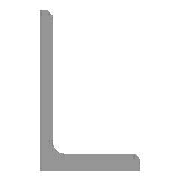
# Autodesk Inventor part: ISO 657-2 - 50x 30x 5-1448.59
Saved by Autodesk Inventor 2023 (Build 270158000, 158)
## iProperties
Created: 2022-09-07
Part Number: ISO 657-2 - 50x 30x 5-1448.59
Material: Steel, Mild
Description: Hot-rolled steel sections - Part 2: Unequal-leg angles
Document SubType Name: Modeling
Standard: ISO 657-2
Designer: Mike
Standard Revision: Hot-rolled steel sections - Part 2: Unequal-leg angles 1989-08-01
Standards Organization: ISO
Language: en-US
Size Designation: 50x 30x 5
Categories: <MemberInstance><Categories><Category DisplayName="Structural Shapes" InternalName="089c4875-fa83-4c05-b084-43b9cc11f5ed" Mnemonic="GRDR"><CategoryParameter DisplayName="Mass per Length Unit" InternalName="0bb95a10-148f-4027-a459-38d7b056702a" Mnemonic="shpmass"/><CategoryParameter DisplayName="Section Area" InternalName="1ff91680-64b0-4202-b9a3-7fd3f94bba3b" Mnemonic="secarea"/><CategoryParameter DisplayName="Radius of Gyration (x)" InternalName="25778675-03e9-40c1-b6a8-4a9ed693320d" Mnemonic="gyrradx"/><CategoryParameter DisplayName="Torsional Rigidity Modulus" InternalName="26c1ec35-5026-4c63-ad0a-751cf684a536" Mnemonic="torrigmod"/><CategoryParameter DisplayName="Distance of the Center of Gravity X-X" InternalName="26c9bdb8-9c79-4b4f-a92e-8e197583c9c4" Mnemonic="grcendistX"/><CategoryParameter DisplayName="Legacy Member ID" InternalName="340afe4f-75d7-48d3-ab7d-943f3c3da468" Mnemonic="LegacyMemberID"/><CategoryParameter DisplayName="Base Length" InternalName="42e34263-8f20-4d0e-ad48-bf1385b87c24" Mnemonic="shplen"/><CategoryParameter DisplayName="Moment of Inertia (y)" InternalName="4b9f58ea-bced-460e-81ea-3d29ca5a49e3" Mnemonic="inermomy"/><CategoryParameter DisplayName="Moment of Inertia (x)" InternalName="4cd780bc-73d7-43ac-917a-579e5cbd684d" Mnemonic="inermomx"/><CategoryParameter DisplayName="Custom Base Point" InternalName="4f1d1b73-316d-484b-a3df-9cbabb16eb77" Mnemonic="shpBasePoint"/><CategoryParameter DisplayName="Shape Height" InternalName="50274e7d-5ac0-4796-92cb-c59e54983c67" Mnemonic="shpheig"/><CategoryParameter DisplayName="Section Module (y)" InternalName="59eaa5e9-d227-48dc-b6c1-6920f96e0f95" Mnemonic="secmody"/><CategoryParameter DisplayName="Section Designation" InternalName="5a64d034-428d-49c8-ba32-7619764de20f" Mnemonic="shpdes"/><CategoryParameter DisplayName="Section Module (x)" InternalName="72cfad18-cf51-4ed4-aaa7-c6b224f8419f" Mnemonic="secmodx"/><CategoryParameter DisplayName="Torsional Section Modulus" InternalName="7c55a8dc-8844-49f9-a867-cc677b30ec9a" Mnemonic="torsecmod"/><CategoryParameter DisplayName="Shape Width" InternalName="7c717d54-a18f-4666-b4d4-573cce22c62c" Mnemonic="shpwdth"/><CategoryParameter DisplayName="Second Shape Thickness" InternalName="9251a8e1-85fd-4e47-af99-afdb762317d9" Mnemonic="shpthick2"/><CategoryParameter DisplayName="FG Authored" InternalName="9c666724-f362-4ea7-ac62-f6a007de5c69" Mnemonic="shpFGAuto"/><CategoryParameter DisplayName="Distance of the Center of Gravity Y-Y" InternalName="bcc4fb17-7af4-436a-8f8c-d0aa3b0248c5" Mnemonic="grcendistY"/><CategoryParameter DisplayName="Radius of Gyration (y)" InternalName="bfa18ebe-1636-4dbe-8d42-b263e0b73184" Mnemonic="gyrrady"/><CategoryParameter DisplayName="Shape Thickness" InternalName="d109cf76-8eb4-42fc-9800-4409734adc67" Mnemonic="shpthick"/><CategoryParameter DisplayName="Coefficient of Shear Displacement" InternalName="de4c90c6-aaa8-468f-a335-6737b311b5d3" Mnemonic="shdispc"/><Category DisplayName="Angles" InternalName="891838e5-6de8-44c9-8a56-cff30cd12e44" Mnemonic="LSHP"><CategoryParameter DisplayName="Shape Width" InternalName="22dbc2a2-e4da-47b4-bbc2-0ed25b88a7c5" Mnemonic="shpwdth"/><CategoryParameter DisplayName="Section Area" InternalName="564a19c2-3cdb-4e61-a3cd-9a0c83be571a" Mnemonic="secarea"/><CategoryParameter DisplayName="Shape Thickness" InternalName="5c12cced-d35f-46db-9d8b-cf5f216ed4b9" Mnemonic="shpthick"/><CategoryParameter DisplayName="Mass per Length Unit" InternalName="c045a850-bfad-4bdf-b14c-077eb4749b94" Mnemonic="shpmass"/><CategoryParameter DisplayName="Radius of Gyration (x)" InternalName="c9deb76c-754a-4e8e-9bc3-4870de9dfe62" Mnemonic="gyrradx"/><CategoryParameter DisplayName="Moment of Inertia (y)" InternalName="d0ed951c-e239-4172-87dd-dbe52d4ee0b6" Mnemonic="inermomy"/><CategoryParameter DisplayName="Second Shape Thickness" InternalName="e2df6b7d-3313-4ea2-80df-fc9eacf16587" Mnemonic="shpthick2"/><CategoryParameter DisplayName="Section Module (x)" InternalName="e378446f-bf2e-4d99-93b0-32dd66c7caa2" Mnemonic="secmodx"/><CategoryParameter DisplayName="Section Module (y)" InternalName="efaf05a1-c4f1-4600-8633-7301da83f3ff" Mnemonic="secmody"/><CategoryParameter DisplayName="Moment of Inertia (x)" InternalName="fd23d820-fefc-47f1-b446-d1304eae789f" Mnemonic="inermomx"/><CategoryParameter DisplayName="Radius of Gyration (y)" InternalName="ff3a8a0d-cdc0-4094-bc22-17f67dad5d84" Mnemonic="gyrrady"/></Category></Category><Category DisplayName="DataType" InternalName="23b78d0f-2648-40c6-8793-ca6db495c9e8" Mnemonic="DATATYPE"><CategoryParameter DisplayName="DisplayName" InternalName="05415f3d-3907-474b-a020-eb9d644f4cf3" Mnemonic="DISPLAYNAME"/><CategoryParameter DisplayName="Standard" InternalName="0c0a119c-1e12-4c84-803f-101930972f5e" Mnemonic="STANDARD"/><CategoryParameter DisplayName="Description" InternalName="13903e3d-64b1-4950-80da-f627842ea37f" Mnemonic="DESCRIPTION"/><CategoryParameter DisplayName="Designation" InternalName="2675968c-4ce5-49e0-a4f5-552d29089031" Mnemonic="DESIGNATION"/><CategoryParameter DisplayName="Default Row" InternalName="2af9ec52-faaa-4026-b378-f9fa4afca842" Mnemonic="DEFAULTROW"/><CategoryParameter DisplayName="Folder Name" InternalName="3f06958e-8713-4116-9be7-ed6184ecc97b" Mnemonic="FOLDERNAME"/><CategoryParameter DisplayName="Revision Guid" InternalName="45a75005-10b1-4dfc-8d6d-dfe629f0b93c" Mnemonic="REVISIONGUID"/><CategoryParameter DisplayName="FileName" InternalName="8b46a4cc-9585-4fed-90c3-899f57e09a73" Mnemonic="FILENAME"/><CategoryParameter DisplayName="StdsOrg" InternalName="8f5914e1-4693-403f-8ab5-d37768198c9d" Mnemonic="STDSORG"/><CategoryParameter DisplayName="Family Version" InternalName="914462f6-6e19-4b14-ba84-155b9680b1d0" Mnemonic="FAMILYREVISION"/><CategoryParameter DisplayName="Standard Revision" InternalName="91d5a463-65c2-4fde-b823-3b7fea5e8e17" Mnemonic="STANDARDREVISION"/><CategoryParameter DisplayName="Member Revision" InternalName="a65d44b9-392f-4f4f-857b-e4b3d54996fe" Mnemonic="MEMBERREVISION"/><CategoryParameter DisplayName="ClipFormat" InternalName="bc51e27b-3422-4e78-93ef-cec197ddf230" Mnemonic="CLIPFORMAT"/><CategoryParameter DisplayName="Manufacturer" InternalName="cd6c7a72-a28a-4e50-99a9-2c7f4e13e5ad" Mnemonic="MANUFACTURER"/><CategoryParameter DisplayName="InternalName" InternalName="cf1d0246-76d9-4b4a-8305-fa0409afb5c1" Mnemonic="INTERNALNAME"/><CategoryParameter DisplayName="IsMetric" InternalName="e2385c5b-1ea4-4823-96a8-8de651266ec3" Mnemonic="ISMETRIC"/><Category DisplayName="Part" InternalName="c0e0b642-3bcb-4cc8-9e80-f96d35c4afa4" Mnemonic="PART"><CategoryParameter DisplayName="Part Number" InternalName="016b6077-bfbe-49bd-92c9-d8d59c39c941" Mnemonic="PARTNUMBER"/><CategoryParameter DisplayName="Stock Number" InternalName="4dba7c1c-e26c-444e-836c-b08b433409a8" Mnemonic="STOCKNUMBER"/><CategoryParameter DisplayName="Material Key" InternalName="5c9a8adb-dd2b-4535-b97f-0a94a95fe41f" Mnemonic="MATERIALKEY"/><CategoryParameter DisplayName="Material" InternalName="818a152a-d3c3-49ca-80ee-df7d91421b8e" Mnemonic="MATERIAL"/></Category></Category><Category DisplayName="LegacyMap" InternalName="cd87c42b-3e48-431e-b5c0-1cbeb14dfe77" Mnemonic="LEGACYMAP"><CategoryParameter DisplayName="unique DA member ID" InternalName="0918ad47-427f-4fed-ae26-24c81c58f590" Mnemonic="DACOOKIE"/><CategoryParameter DisplayName="Merge11 ID" InternalName="0ee8fb18-e2ed-4f39-96f6-1f4b5f50aa71" Mnemonic="MERGE11"/><CategoryParameter DisplayName="unique CC member ID" InternalName="5193edd4-b2b0-4ab4-9d54-de900eee34e0" Mnemonic="CCCOOKIE"/><CategoryParameter DisplayName="Split ID" InternalName="72b5c83c-be7f-45c4-ae51-9160ea6deb26" Mnemonic="SPLIT"/><CategoryParameter DisplayName="MemberID" InternalName="8e5e0294-fc51-4c8f-b3d7-003dc5ed94f6" Mnemonic="MEMBERID"/><CategoryParameter DisplayName="CatalogName" InternalName="d99d1e27-aa94-4de2-af4c-c348882a6f4f" Mnemonic="CATALOGNAME"/><CategoryParameter DisplayName="FamilyNumber" InternalName="e705e1f4-09cb-413e-91f9-551b4188271e" Mnemonic="FAMILYNUMBER"/></Category></Categories><FamilyTemplate Id="N425545"><FamilyTemplateParameters><FamilyTemplateParameter ObjectType="kUserParameterObject" ValueType="xs:double" Id="1" ObjectReferenceKey="ParH"/><FamilyTemplateParameter ObjectType="kUserParameterObject" ValueType="xs:double" Id="2" ObjectReferenceKey="b"/><FamilyTemplateParameter ObjectType="kUserParameterObject" ValueType="xs:double" Id="3" ObjectReferenceKey="ParT"/><FamilyTemplateParameter ObjectType="kUserParameterObject" ValueType="xs:double" Id="4" ObjectReferenceKey="B_L"/><FamilyTemplateParameter ObjectType="kUserParameterObject" ValueType="xs:double" Id="6" ObjectReferenceKey="R"/><FamilyTemplateParameter ObjectType="kUserParameterObject" ValueType="xs:double" Id="7" ObjectReferenceKey="R1"/><FamilyTemplateParameter ObjectType="kUserParameterObject" ValueType="xs:double" Id="8" ObjectReferenceKey="ex"/><FamilyTemplateParameter ObjectType="kUserParameterObject" ValueType="xs:double" Id="9" ObjectReferenceKey="ey"/><FamilyTemplateParameter ObjectType="kPropertyObject" ValueType="xs:string" Id="100" ObjectReferenceKey="{32853F0F-3444-11d1-9E93-0060B03C1CA6}" SubObjectId="52"/><FamilyTemplateParameter ObjectType="kPropertyObject" ValueType="xs:string" Id="105" ObjectReferenceKey="{32853F0F-3444-11d1-9E93-0060B03C1CA6}" SubObjectId="5"/><FamilyTemplateParameter ObjectType="kPartComponentDefinitionObject" ValueType="xs:string" Id="110" SubObjectId="Material"/><FamilyTemplateParameter ObjectType="kPropertyObject" ValueType="xs:string" Id="112" ObjectReferenceKey="{32853F0F-3444-11d1-9E93-0060B03C1CA6}" SubObjectId="55"/></FamilyTemplateParameters></FamilyTemplate><CategoryParameterMap><ParamToTemplateMap><ParamToTemplate CategoryParameter="//CategoryParameter[@InternalName='05415f3d-3907-474b-a020-eb9d644f4cf3']" ConstantValue="ISO 657-2"/><ParamToTemplate CategoryParameter="//CategoryParameter[@InternalName='cf1d0246-76d9-4b4a-8305-fa0409afb5c1']" ConstantValue="F30FCBF5-6888-4DB7-AC61-FFBE56B72853"/><ParamToTemplate CategoryParameter="//CategoryParameter[@InternalName='3f06958e-8713-4116-9be7-ed6184ecc97b']" ConstantValue="ISO 657-2(1)"/><ParamToTemplate CategoryParameter="//CategoryParameter[@InternalName='914462f6-6e19-4b14-ba84-155b9680b1d0']" ConstantValue="10"/><ParamToTemplate CategoryParameter="//CategoryParameter[@InternalName='bc51e27b-3422-4e78-93ef-cec197ddf230']" ConstantValue="CF_INVENTOR.STDPARTS"/><ParamToTemplate CategoryParameter="//CategoryParameter[@InternalName='e2385c5b-1ea4-4823-96a8-8de651266ec3']" ConstantValue="true"/><ParamToTemplate CategoryParameter="//CategoryParameter[@InternalName='13903e3d-64b1-4950-80da-f627842ea37f']" ConstantValue="Hot-rolled steel sections - Part 2: Unequal-leg angles"/><ParamToTemplate CategoryParameter="//CategoryParameter[@InternalName='8f5914e1-4693-403f-8ab5-d37768198c9d']" ConstantValue="ISO"/><ParamToTemplate CategoryParameter="//CategoryParameter[@InternalName='0c0a119c-1e12-4c84-803f-101930972f5e']" ConstantValue="ISO 657-2"/><ParamToTemplate CategoryParameter="//CategoryParameter[@InternalName='cd6c7a72-a28a-4e50-99a9-2c7f4e13e5ad']" TemplateParameter="104"/><ParamToTemplate CategoryParameter="//CategoryParameter[@InternalName='91d5a463-65c2-4fde-b823-3b7fea5e8e17']" ConstantValue="Hot-rolled steel sections - Part 2: Unequal-leg angles 1989-08-01"/><ParamToTemplate CategoryParameter="//CategoryParameter[@InternalName='45a75005-10b1-4dfc-8d6d-dfe629f0b93c']" ConstantValue="9f63e30b-fb1f-4f85-8ad4-df521d37c4ef"/><ParamToTemplate CategoryParameter="//CategoryParameter[@InternalName='2af9ec52-faaa-4026-b378-f9fa4afca842']" ConstantValue="10"/><ParamToTemplate CategoryParameter="//CategoryParameter[@InternalName='9c666724-f362-4ea7-ac62-f6a007de5c69']" ConstantValue="1"/><ParamToTemplate CategoryParameter="//CategoryParameter[@InternalName='8b46a4cc-9585-4fed-90c3-899f57e09a73']" ConstantValue="ISO 657-2 - 50x 30x 5-1(1)"/><ParamToTemplate CategoryParameter="//CategoryParameter[@InternalName='a65d44b9-392f-4f4f-857b-e4b3d54996fe']" ConstantValue="FD8DB589-BC97-47AD-B44D-88836A288CB3"/><ParamToTemplate CategoryParameter="//CategoryParameter[@InternalName='fd23d820-fefc-47f1-b446-d1304eae789f']" ConstantValue="93600"/><ParamToTemplate CategoryParameter="//CategoryParameter[@InternalName='d0ed951c-e239-4172-87dd-dbe52d4ee0b6']" ConstantValue="25100"/><ParamToTemplate CategoryParameter="//CategoryParameter[@InternalName='e378446f-bf2e-4d99-93b0-32dd66c7caa2']" ConstantValue="2860"/><ParamToTemplate CategoryParameter="//CategoryParameter[@InternalName='efaf05a1-c4f1-4600-8633-7301da83f3ff']" ConstantValue="1110"/><ParamToTemplate CategoryParameter="//CategoryParameter[@InternalName='564a19c2-3cdb-4e61-a3cd-9a0c83be571a']" ConstantValue="378"/><ParamToTemplate CategoryParameter="//CategoryParameter[@InternalName='7c55a8dc-8844-49f9-a867-cc677b30ec9a']" ConstantValue="618.75"/><ParamToTemplate CategoryParameter="//CategoryParameter[@InternalName='26c1ec35-5026-4c63-ad0a-751cf684a536']" ConstantValue="3093.75"/><ParamToTemplate CategoryParameter="//CategoryParameter[@InternalName='de4c90c6-aaa8-468f-a335-6737b311b5d3']" ConstantValue="2.1"/><ParamToTemplate CategoryParameter="//CategoryParameter[@InternalName='c9deb76c-754a-4e8e-9bc3-4870de9dfe62']" ConstantValue="15.7"/><ParamToTemplate CategoryParameter="//CategoryParameter[@InternalName='ff3a8a0d-cdc0-4094-bc22-17f67dad5d84']" ConstantValue="8.16"/><ParamToTemplate CategoryParameter="//CategoryParameter[@InternalName='0918ad47-427f-4fed-ae26-24c81c58f590']" ConstantValue="*AFN~N425545~L50x30x5-25000*ISO~N425545~L50x30x5-25000*"/><ParamToTemplate CategoryParameter="//CategoryParameter[@InternalName='0ee8fb18-e2ed-4f39-96f6-1f4b5f50aa71']" ConstantValue="^df3a0830-ff12-4aeb-8c97-2ce33836734a^2693A280-8F42-485B-B5CC-E84E51971F05^"/><ParamToTemplate CategoryParameter="//CategoryParameter[@InternalName='42e34263-8f20-4d0e-ad48-bf1385b87c24']" TemplateParameter="4"/><ParamToTemplate CategoryParameter="//CategoryParameter[@InternalName='2675968c-4ce5-49e0-a4f5-552d29089031']" TemplateParameter="100"/><ParamToTemplate CategoryParameter="//CategoryParameter[@InternalName='818a152a-d3c3-49ca-80ee-df7d91421b8e']" TemplateParameter="110"/><ParamToTemplate CategoryParameter="//CategoryParameter[@InternalName='016b6077-bfbe-49bd-92c9-d8d59c39c941']" TemplateParameter="105"/><ParamToTemplate CategoryParameter="//CategoryParameter[@InternalName='4dba7c1c-e26c-444e-836c-b08b433409a8']" TemplateParameter="112"/><ParamToTemplate CategoryParameter="//CategoryParameter[@InternalName='26c9bdb8-9c79-4b4f-a92e-8e197583c9c4']" TemplateParameter="8"/><ParamToTemplate CategoryParameter="//CategoryParameter[@InternalName='bcc4fb17-7af4-436a-8f8c-d0aa3b0248c5']" TemplateParameter="9"/></ParamToTemplateMap></CategoryParameterMap></MemberInstance>
Stock Number: 50x 30x 5
Density: 7.85 g/cm^3
Appearance: Semi-Polished
IsCustomPart: 1
_CCFamilyMember: 70
_CCFamilyDisplayName: ISO 657-2 - Hot-rolled steel sections - Part 2: Unequal-leg angles
_FrameMemberDoc: Frame Member File
_Version: 25.0.0
_GetPNFromCC: 1
Author: Mike
G_L: 1448.586 mm
G_W: 30.000 mm
G_H: 50.000 mm
+C16140E9-773F-483F-8440-83743AC13685+CUTDETAIL1: Miter 45.00 deg
+0C277CC3-ED62-4754-A70B-EEED72D871A1+CUTDETAIL2: Miter 45.00 deg
Autodesk Inventor part; units mm, degrees
ref_plane "Start Plane" through (0, 0, -24.2929) normal (0, 0, 1) x (1, 0, 0)
ref_plane "End Plane" through (0, 0, 1424.2929) normal (0, 0, 1) x (1, 0, 0)
sketch "Sketch" plane through (0, 0, 0) normal (0, 0, 1) x (1, 0, 0)
  line L0 (-2.41, 28.7) -> (-2.41, -7.3)
  line L1 (-7.41, 32.7) -> (-6.41, 32.7)
  line L2 (-7.41, -17.3) -> (-7.41, 32.7)
  line L3 (22.59, -17.3) -> (-7.41, -17.3)
  line L4 (22.59, -16.3) -> (22.59, -17.3)
  line L5 (2.59, -12.3) -> (18.59, -12.3)
  arc A0 (-2.41, -7.3) -> (2.59, -12.3) centre (2.59, -7.3) ccw
  arc A1 (-2.41, 28.7) -> (-6.41, 32.7) centre (-6.41, 28.7) ccw
  arc A2 (22.59, -16.3) -> (18.59, -12.3) centre (18.59, -16.3) ccw
  line L6 (0, 43.6941) -> (0, -27.4657) construction
  line L7 (-13.5757, 0) -> (29.5841, 0) construction
  point P0 (-2.41, 32.7)
  point P1 (-2.41, -12.3)
  point P2 (22.59, -12.3)
  dimension "d4" = 30
  dimension "d6" = 50
  dimension "d8" = 5
  dimension "d10" = 5
  dimension "d17" = 5
  dimension "d18" = 4
  dimension "d19" = 17.3
  dimension "d20" = 7.41
  constraints: 12 end point, 6 point on circle, 6 point on line, 6 tangent, 3 centre point, 3 horizontal, 3 vertical, 1 equal radius
  measures "d4" distance of L3.start L2.start
  measures "d6" distance of L2.start L1.start
  measures "d8" distance of point (22.59, -12.3) L3.start
  measures "d10" distance of L1.start point (-2.41, 32.7)
  measures "d17" radius of A0
  measures "d18" radius of A1
  measures "d19" distance between parallel lines of L7 L3
  measures "d20" distance between parallel lines of L2 L6
extrude "Body" add sketch "Sketch" along normal up to surface (1448.5858 mm away) from surface at -24.2929
sketch "Sketch3" plane through (0, 0, 0) normal (0, 0, 1) x (1, 0, 0)
  line L0 (0, 0) -> (10, 0)
ref_plane "Work Plane10" through (0, 0, 0) normal (0, -1, 0) x (1, 0, 0)
sketch "Sketch4" plane through (0, 0, 0) normal (0, -1, 0) x (1, 0, 0)
  line L0 (-2, -24.2929) -> (12, -24.2929)
  line L1 (-2, 1424.2929) -> (12, 1424.2929)
  dimension "d24" = 1448.5858
  measures "d24" distance between parallel lines of L0 L1
ref_plane "Work Plane11" through (7.59, -17.6536, 1424.6464) normal (0, 0.7071, 0.7071) x (1, 0, 0)
split "Split1" plane through (7.59, -17.6536, 1424.6464) removes the side toward (0, 0.7071, 0.7071)
ref_plane "Work Plane12" through (7.59, -17.6536, -24.6464) normal (0, 0.7071, -0.7071) x (1, 0, 0)
split "Split2" plane through (7.59, -17.6536, -24.6464) removes the side toward (0, 0.7071, -0.7071)
equation "\"d4\" = b"
equation "\"d6\" = ParH"
equation "\"d8\" = ParT"
equation "\"d10\" = ParT"
equation "\"d17\" = R"
equation "\"d18\" = R1"
equation "\"d19\" = ex"
equation "\"d20\" = ey"
equation "\"d11\" = G_L"
equation "\"b\" = 30"
equation "\"ParT\" = 5"
equation "\"R1\" = 4"
equation "\"G_L\" = d24"
equation "\"ParH\" = 50"
equation "\"R\" = 5"
equation "\"ey\" = 7.41"
equation "\"ex\" = 17.3"
equation "\"G_OFFSET_START\" = 24.29289"
equation "\"G_OFFSET_END\" = 24.29289"
equation "\"d21\" = -G_OFFSET_START"
equation "\"d22\" = G_OFFSET_END + B_L"
equation "\"B_L\" = 1400"
body "Solid1"
